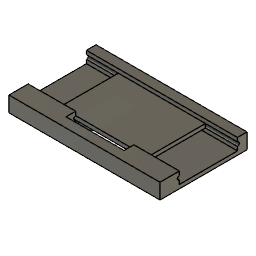
reaction wheel pendulum (Autodesk Fusion 360 archive; units mm, degrees)
design "computer stand"
Autodesk Fusion 360 part; units mm, degrees
(part 1 of 2)
sketch "スケッチ1" plane through (0, 0, 0) normal (0, 0, 1) x (1, 0, 0)
  line L0 (0, 0) -> (-50, 0)
  line L1 (-50, 0) -> (-50, -35)
  line L2 (-50, -35) -> (0, -35)
  line L3 (0, -35) -> (0, 0)
  line L4 (-65, 5) -> (15, 5)
  line L5 (15, 5) -> (15, -40)
  line L6 (15, -40) -> (-65, -40)
  line L7 (-65, -40) -> (-65, 5)
  constraint horizontal L0
  constraint vertical L1
  constraint horizontal L2
  constraint vertical L3
  constraint coincident L0.start L3.end
  constraint horizontal L4
  constraint vertical L5
  constraint horizontal L6
  constraint vertical L7
extrude "押し出し1" add sketch "スケッチ1" against normal blind 5 contours L0 L1 L2 L3 makes body 1
extrude "押し出し2" add sketch "スケッチ1" along normal blind 5 contours L0 L1 L2 L3 | L4 L5 L6 L7 bodies 1
sketch "スケッチ2" plane through (0, 0, 5) normal (0, 0, 1) x (-1, 0, 0)
  line L0 (65, 40) -> (-15, 40)
  line L1 (-15, 40) -> (-15, -5)
  line L2 (-15, -5) -> (65, -5)
  line L3 (65, -5) -> (65, 40)
  line L4 (-15, 0) -> (65, 0)
  line L5 (65, 0) -> (65, 30)
  line L6 (65, 30) -> (-15, 30)
  line L7 (-15, 30) -> (-15, 0)
  constraint horizontal L4
  constraint vertical L5
  constraint horizontal L6
  constraint vertical L7
  constraint coincident L3 L5.end
  constraint coincident L1 L4.start
extrude "押し出し3" cut sketch "スケッチ2" against normal blind 3 contours L1 L3 L4 L5 L6 L7 bodies 1
sketch "スケッチ3" plane through (0, 0, -5) normal (0, 0, -1) x (1, 0, 0)
  line L0 (0, 0) -> (0, 35)
  line L1 (0, 35) -> (-50, 35)
  line L2 (-50, 35) -> (-50, 0)
  line L3 (-50, 0) -> (0, 0)
  line L4 (-10, 0) -> (-40, 0)
  line L5 (-40, 0) -> (-40, 35)
  line L6 (-40, 35) -> (-10, 35)
  line L7 (-10, 35) -> (-10, 0)
  constraint horizontal L4
  constraint vertical L5
  constraint horizontal L6
  constraint vertical L7
  constraint coincident L1 L5.end
  constraint coincident L3 L4.start
extrude "押し出し4" cut sketch "スケッチ3" against normal blind 10 contours L1 L3 L4 L5 L6 L7 bodies 1
extrude "押し出し5" add 2 faces at (-38.3333, 3.3333, 5) (-56.6667, -35, 5) along direction (0, 0, 1) blind 3 on bodies 1 bodies 1
sketch "スケッチ4" plane through (-65, 0, 0) normal (-1, 0, 0) x (0, -1, 0)
  line L0 (0, 2) -> (0, 8)
  line L1 (0, 8) -> (-5, 8)
  line L2 (-5, 8) -> (-5, 0)
  line L3 (-5, 0) -> (40, 0)
  line L4 (40, 0) -> (40, 8)
  line L5 (40, 8) -> (30, 8)
  line L6 (30, 8) -> (30, 2)
  line L7 (30, 2) -> (0, 2)
  line L8 (0, 5) -> (30, 5)
  line L9 (0, 4) -> (30, 4)
  arc A0 (30, 4) -> (30, 6) centre (30, 5) ccw
  line L10 (30, 6) -> (0, 6)
  arc A1 (0, 6) -> (0, 4) centre (0, 5) ccw
  line L11 (0, 5) -> (30, 5) construction
  constraint midpoint L0 L8.start
  constraint midpoint L6 L8.end
  constraint tangent L9 A0
  constraint tangent A0 L10
  constraint parallel L9 L10
  constraint tangent L10 A1
  constraint tangent L9 A1
  constraint coincident L8.end A0.centre
  constraint perpendicular L6 L11
  constraint coincident L8.start A1.centre
extrude "押し出し6" cut sketch "スケッチ4" against normal blind 80 contours L0 A1 | L6 A0 bodies 1
sketch "スケッチ5" plane through (0, 0, -5) normal (0, 0, -1) x (1, 0, 0)
  line L0 (-40, 0) -> (-40, 35)
  line L1 (-40, 35) -> (-50, 35)
  line L2 (-50, 35) -> (-50, 0)
  line L3 (-50, 0) -> (-40, 0)
extrude "押し出し7" cut 1 faces at (-65, -36.9916, 4.2592) along direction (1, 0, 0) blind 1 on bodies 1 bodies 1
extrude "押し出し8" cut 1 faces at (-64, -36.9916, 4.2592) along direction (1, 0, 0) blind 1 on bodies 1 bodies 1
extrude "押し出し9" cut 1 faces at (15, -36.9916, 4.2592) along direction (-1, 0, 0) blind 1 on bodies 1 bodies 1
extrude "押し出し10" add 1 faces at (-63, -36.9916, 4.2592) along direction (-1, 0, 0) blind 0.5 on bodies 1 bodies 1
extrude "押し出し11" cut 1 faces at (14, -36.9916, 4.2592) along direction (-1, 0, 0) blind 0.5 on bodies 1 bodies 1
extrude "押し出し12" cut 1 faces at (0, -23.3333, -3.3333) along direction (-1, 0, 0) blind 0.25 on bodies 1 bodies 1
extrude "押し出し13" cut 1 faces at (-50, -11.6667, -3.3333) along direction (1, 0, 0) blind 0.25 on bodies 1 bodies 1
extrude "押し出し14" add 1 faces at (-63.5, -36.9916, 4.2592) along direction (-1, 0, 0) blind 1 on bodies 1 bodies 1
sketch "スケッチ6" plane through (-64.5, 0, 0) normal (-1, 0, 0) x (0, -1, 0)
  arc A0 (0, 6) -> (0, 4) centre (0, 5) ccw
  line L0 (0, 6) -> (0, 8)
  line L1 (0, 8) -> (-5, 8)
  line L2 (-5, 8) -> (-5, 0)
  line L3 (-5, 0) -> (40, 0)
  line L4 (40, 0) -> (40, 8)
  line L5 (40, 8) -> (30, 8)
  line L6 (30, 8) -> (30, 6)
  arc A1 (30, 4) -> (30, 6) centre (30, 5) ccw
  line L7 (30, 4) -> (30, 2)
  line L8 (30, 2) -> (0, 2)
  line L9 (0, 2) -> (0, 4)
  line L10 (0, 6) -> (30, 6)
  line L11 (30, 6) -> (30, 4)
  line L12 (30, 4) -> (0, 4)
  line L13 (0, 4) -> (0, 6)
  line L14 (0, 6) -> (30, 4) construction
  line L15 (30, 6) -> (0, 4) construction
  point P0 (15, 5)
  constraint horizontal L10
  constraint perpendicular L10 L11
  constraint parallel L10 L12
  constraint parallel L11 L13
  constraint coincident L14 P0
  constraint coincident L15 P0
  constraint coincident A0.start L0.start
  constraint coincident A1.start L7.start
extrude "押し出し15" add sketch "スケッチ6" against normal blind 78 separate body contours L10 L11 L12 L13 makes body 2
sketch "スケッチ7" plane through (0, 0, 6) normal (0, 0, 1) x (-1, 0, 0)
  line L0 (64.5, 0) -> (64.5, 30)
  line L1 (64.5, 30) -> (-13.5, 30)
  line L2 (-13.5, 30) -> (-13.5, 0)
  line L3 (-13.5, 0) -> (64.5, 0)
  line L4 (3, 30) -> (48, 30)
  line L5 (48, 30) -> (48, 0)
  line L6 (48, 0) -> (3, 0)
  line L7 (3, 0) -> (3, 30)
  line L8 (3, 30) -> (48, 0) construction
  line L9 (48, 30) -> (3, 0) construction
  point P0 (25.5, 15)
  dimension "d31" = 39
  dimension "d32" = 45
  constraint horizontal L4
  constraint perpendicular L4 L5
  constraint parallel L4 L6
  constraint parallel L5 L7
  constraint coincident L8 P0
  constraint coincident L9 P0
  constraint coincident L1 L4.start
  constraint coincident L3 L6.end
  measures "d31" distance of L2 P0
  measures "d32" distance of L4.start L4.end
extrude "押し出し16" cut sketch "スケッチ7" against normal blind 2 contours L0 L1 L3 L5 | L1 L2 L3 L7 bodies 2

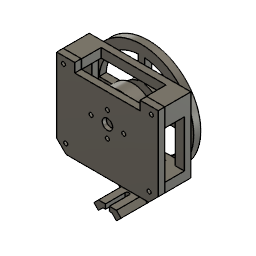
design "モータ取り付け台"
Autodesk Fusion 360 part; units mm, degrees
sketch "スケッチ1" plane through (0, 0, 0) normal (0, 0, 1) x (1, 0, 0)
  line L0 (-38.8909, 38.8909) -> (0, 0)
  line L1 (0, 0) -> (38.8909, 38.8909)
  line L2 (38.8909, 38.8909) -> (-38.8909, 38.8909) construction
  line L3 (0, 38.8909) -> (0, 0) construction
  line L4 (-24.5921, 31.6632) -> (-3.3789, 10.45)
  line L5 (-3.3789, 10.45) -> (3.3789, 10.45)
  line L6 (3.3789, 10.45) -> (24.5921, 31.6632)
  line L7 (24.5921, 31.6632) -> (24.5921, 38.8909)
  line L8 (-24.5921, 38.8909) -> (-24.5921, 31.6632)
  line L9 (-24.5921, 38.8909) -> (24.5921, 38.8909)
  line L10 (-38.8909, 38.8909) -> (-38.8909, 45.9909)
  line L11 (-31.8909, 45.9909) -> (31.8909, 45.9909)
  line L12 (38.8909, 45.9909) -> (38.8909, 38.8909)
  line L13 (31.8909, 45.9909) -> (-31.8909, 45.9909)
  line L14 (-38.8909, 45.9909) -> (-38.8909, 95.9909)
  line L15 (-38.8909, 95.9909) -> (38.8909, 95.9909)
  line L16 (38.8909, 95.9909) -> (38.8909, 45.9909)
  line L17 (38.8909, 45.9909) -> (-38.8909, 95.9909) construction
  line L18 (-38.8909, 45.9909) -> (38.8909, 95.9909) construction
  line L19 (-31.8909, 45.9909) -> (-31.8909, 81.9198)
  line L20 (-24.8198, 88.9909) -> (24.8198, 88.9909)
  line L21 (31.8909, 81.9198) -> (31.8909, 45.9909)
  line L22 (-24.8198, 88.9909) -> (-31.8909, 81.9198)
  line L23 (24.8198, 88.9909) -> (31.8909, 81.9198)
  point P0 (0, 70.9909)
  point P1 (0, 70.9909)
  dimension "d1" = 55
  dimension "d3" = 55
  dimension "d4" = 5
  dimension "d5" = 5
  dimension "d6" = 30
  dimension "d7" = 30
  dimension "d8" = 10.45
  dimension "d9" = 7.1
  dimension "d10" = 50
  dimension "d11" = 7
  dimension "d13" = 45
  dimension "d14" = 45
  dimension "d15" = 10
  dimension "d16" = 10
  dimension "d17" = 7
  dimension "d18" = 7
  dimension "d19" = 57.1
  dimension "d20" = 7.1
  constraint coincident L0.end L1.start
  constraint horizontal L2
  constraint midpoint L2 L3.start
  constraint perpendicular L3 L5
  constraint parallel L0 L4
  constraint parallel L1 L6
  constraint perpendicular L0 L1
  constraint vertical L8
  constraint vertical L7
  constraint coincident L2 L8.start
  constraint coincident L2 L7.end
  constraint coincident L0.start L2.end
  constraint horizontal L11
  constraint vertical L10
  constraint vertical L12
  constraint horizontal L13
  constraint perpendicular L13 L14
  constraint parallel L13 L15
  constraint parallel L14 L16
  constraint coincident L17 P1
  constraint coincident L18 P1
  constraint coincident L10.end L14.start
  constraint coincident P1 P0
  measures "d1" distance of L0.end L1.end
  measures "d3" distance of L0.start L0.end
  measures "d4" distance of L1 L6
  measures "d5" distance of L0 L4
  measures "d6" distance of L5.end L6.end
  measures "d7" distance of L4.start L4.end
  measures "d8" distance of L0.end L5
  measures "d9" distance of L9 L11
  measures "d10" distance of L12.start L15.end
  measures "d11" distance of L16 L21
  measures "d13" angle of L20 L22
  measures "d14" angle of L20 L23
  measures "d15" distance of L20.start L19.end
  measures "d16" distance of L20.end L21.start
  measures "d17" distance of L15 L20
  measures "d18" distance of L14 L19
  measures "d19" distance of L9 L15
  measures "d20" distance of L0.start L10.end
extrude "押し出し1" add sketch "スケッチ1" along normal mid plane 5 makes body 1
sketch "スケッチ2" plane through (0, 0, 2.5) normal (0, 0, 1) x (1, 0, 0)
  line L0 (-31.8909, 81.9198) -> (-24.8198, 88.9909)
  line L1 (-24.8198, 88.9909) -> (24.8198, 88.9909)
  line L2 (24.8198, 88.9909) -> (31.8909, 81.9198)
  line L3 (31.8909, 81.9198) -> (31.8909, 45.9909)
  line L4 (31.8909, 45.9909) -> (-31.8909, 45.9909)
  line L5 (-31.8909, 45.9909) -> (-31.8909, 81.9198)
  line L6 (-3.3789, 10.45) -> (-24.5921, 31.6632)
  line L7 (-24.5921, 31.6632) -> (-24.5921, 38.8909)
  line L8 (-24.5921, 38.8909) -> (24.5921, 38.8909)
  line L9 (24.5921, 38.8909) -> (24.5921, 31.6632)
  line L10 (24.5921, 31.6632) -> (3.3789, 10.45)
  line L11 (3.3789, 10.45) -> (-3.3789, 10.45)
  line L12 (-38.8909, 38.8909) -> (0, 0)
  line L13 (0, 0) -> (38.8909, 38.8909)
  line L14 (38.8909, 38.8909) -> (38.8909, 95.9909)
  line L15 (38.8909, 95.9909) -> (-38.8909, 95.9909)
  line L16 (-38.8909, 95.9909) -> (-38.8909, 38.8909)
  line L17 (-24.8198, 95.9909) -> (-24.8198, 88.9909)
  line L18 (-24.8198, 88.9909) -> (-31.8909, 81.9198)
  line L19 (-31.8909, 81.9198) -> (-38.8909, 81.9198)
  line L20 (-38.8909, 81.9198) -> (-38.8909, 95.9909)
  line L21 (-38.8909, 95.9909) -> (-24.8198, 95.9909)
  line L22 (24.8198, 95.9909) -> (24.8198, 88.9909)
  line L23 (24.8198, 88.9909) -> (31.8909, 81.9198)
  line L24 (31.8909, 81.9198) -> (38.8909, 81.9198)
  line L25 (38.8909, 81.9198) -> (38.8909, 95.9909)
  line L26 (38.8909, 95.9909) -> (24.8198, 95.9909)
  line L27 (-24.5921, 45.9909) -> (-24.5921, 31.6632)
  line L28 (-24.5921, 31.6632) -> (-31.6632, 31.6632)
  line L29 (-31.6632, 31.6632) -> (-38.8909, 38.8909)
  line L30 (-38.8909, 38.8909) -> (-38.8909, 45.9909)
  line L31 (-38.8909, 45.9909) -> (-24.5921, 45.9909)
  line L32 (24.5921, 45.9909) -> (24.5921, 31.6632)
  line L33 (24.5921, 31.6632) -> (31.6632, 31.6632)
  line L34 (31.6632, 31.6632) -> (38.8909, 38.8909)
  line L35 (38.8909, 38.8909) -> (38.8909, 45.9909)
  line L36 (38.8909, 45.9909) -> (24.5921, 45.9909)
  line L37 (-3.3789, 10.45) -> (-6.9145, 6.9145)
  line L38 (-6.9145, 6.9145) -> (0, 0)
  line L39 (0, 0) -> (6.9145, 6.9145)
  line L40 (6.9145, 6.9145) -> (3.3789, 10.45)
  line L41 (3.3789, 10.45) -> (-3.3789, 10.45)
  constraint coincident L15 L17.start
  constraint coincident L0.end L1.start
  constraint perpendicular L1 L17
  constraint coincident L0.start L5.end
  constraint coincident L16 L19.end
  constraint perpendicular L16 L19
  constraint coincident L15.end L16.start
  constraint coincident L15 L22.start
  constraint coincident L1.end L2.start
  constraint coincident L2.end L3.start
  constraint coincident L14 L24.end
  constraint perpendicular L14 L24
  constraint coincident L14.end L15.start
  constraint vertical L22
  constraint coincident L4 L27.start
  constraint coincident L6.end L7.start
  constraint coincident L12 L28.end
  constraint perpendicular L27 L28
  constraint vertical L27
  constraint coincident L16 L30.end
  constraint coincident L12.start L16.end
  constraint horizontal L31
  constraint vertical L32
  constraint perpendicular L32 L33
  constraint perpendicular L33 L35
  constraint coincident L4 L32.start
  constraint coincident L9.end L10.start
  constraint coincident L13 L33.end
  constraint coincident L14 L35.end
  constraint coincident L13.end L14.start
  constraint horizontal L36
  constraint coincident L6.start L11.end
  constraint coincident L12 L37.end
  constraint perpendicular L12 L37
  constraint perpendicular L12 L39
  constraint coincident L10.end L11.start
  constraint coincident L13 L39.end
  constraint coincident L12.end L13.start
  constraint perpendicular L13 L40
extrude "押し出し2" add sketch "スケッチ2" along normal blind 15 contours L0 L15 L16 L17 L18 L19 L20 L21 | L4 L7 L12 L16 L27 L28 L29 L30 L31 | L2 L14 L15 L22 L23 L24 L25 L26 | L4 L9 L13 L14 L32 L33 L34 L35 L36 bodies 1
extrude "押し出し3" add sketch "スケッチ2" along normal blind 60 contours L11 L12 L13 L37 L38 L39 L40 L41 bodies 1
sketch "スケッチ3" plane through (0, 0, -2.5) normal (0, 0, -1) x (-1, 0, 0)
  line L0 (24.8198, 88.9909) -> (31.8909, 81.9198)
  line L1 (31.8909, 81.9198) -> (31.8909, 45.9909)
  line L2 (31.8909, 45.9909) -> (-31.8909, 45.9909)
  line L3 (-31.8909, 45.9909) -> (-31.8909, 81.9198)
  line L4 (-31.8909, 81.9198) -> (-24.8198, 88.9909)
  line L5 (-24.8198, 88.9909) -> (24.8198, 88.9909)
  line L6 (24.5921, 31.6632) -> (3.3789, 10.45)
  line L7 (3.3789, 10.45) -> (-3.3789, 10.45)
  line L8 (-3.3789, 10.45) -> (-24.5921, 31.6632)
  line L9 (-24.5921, 31.6632) -> (-24.5921, 38.8909)
  line L10 (-24.5921, 38.8909) -> (24.5921, 38.8909)
  line L11 (24.5921, 38.8909) -> (24.5921, 31.6632)
  line L12 (0, 0) -> (38.8909, 38.8909)
  line L13 (38.8909, 38.8909) -> (38.8909, 95.9909)
  line L14 (38.8909, 95.9909) -> (-38.8909, 95.9909)
  line L15 (-38.8909, 95.9909) -> (-38.8909, 38.8909)
  line L16 (-38.8909, 38.8909) -> (0, 0)
  line L17 (-38.8909, 95.9909) -> (-28.3553, 85.4553) construction
  line L18 (38.8909, 95.9909) -> (28.3553, 85.4553) construction
  circle A0 centre (-33.6231, 90.7231) radius 3.5
  circle A1 centre (33.6231, 90.7231) radius 3.5
  circle A2 centre (-31.8909, 38.8909) radius 3.5
  circle A3 centre (31.8909, 38.8909) radius 3.5
  line L19 (-24.5921, 38.8909) -> (-38.8909, 38.8909) construction
  line L20 (-31.8909, 45.9909) -> (-31.8909, 31.8909) construction
  line L21 (24.5921, 38.8909) -> (38.8909, 38.8909) construction
  line L22 (31.8909, 45.9909) -> (31.8909, 31.8909) construction
  circle A4 centre (-31.8909, 38.8909) radius 1.5
  circle A5 centre (31.8909, 38.8909) radius 1.5
  circle A6 centre (33.6231, 90.7231) radius 1.5
  circle A7 centre (-33.6231, 90.7231) radius 1.5
  dimension "d27" = 7
  dimension "d28" = 7
  dimension "d29" = 7
  dimension "d30" = 7
  dimension "d31" = 3
  dimension "d32" = 3
  dimension "d33" = 3
  dimension "d34" = 3
  constraint coincident L14.end L15.start
  constraint midpoint L4 L17.end
  constraint coincident L13.end L14.start
  constraint midpoint L0 L18.end
  constraint midpoint L17 A0.centre
  constraint midpoint L18 A1.centre
  constraint coincident L9.end L10.start
  constraint coincident L15.end L16.start
  constraint coincident L2.end L3.start
  constraint coincident L16 L20.end
  constraint perpendicular L19 L20
  constraint coincident A2.centre L19
  constraint coincident A2.centre L20
  constraint coincident L10.end L11.start
  constraint coincident L12.end L13.start
  constraint coincident L1.end L2.start
  constraint coincident L12 L22.end
  constraint perpendicular L21 L22
  constraint coincident A3.centre L22
  constraint coincident A3.centre L21
  constraint concentric A2 A4
  constraint concentric A3 A5
  constraint concentric A1 A6
  constraint concentric A0 A7
  measures "d27" diameter of A0
  measures "d28" diameter of A1
  measures "d29" diameter of A2
  measures "d30" diameter of A3
  measures "d31" diameter of A4
  measures "d32" diameter of A5
  measures "d33" diameter of A6
  measures "d34" diameter of A7
extrude "押し出し4" cut sketch "スケッチ3" against normal blind 25 contours A4 | A5 | A6 | A7 bodies 1
extrude "押し出し7" cut 1 faces at (0, 6.9667, 62.5) along direction (0, 0, -1) blind 65 on bodies 1 bodies 1
sketch "スケッチ8" plane through (0, 0, 2.5) normal (0, 0, 1) x (1, 0, 0)
  line L0 (-6.9145, 6.9145) -> (-3.3789, 10.45)
  line L1 (-3.3789, 10.45) -> (-24.5921, 31.6632)
  line L2 (-24.5921, 31.6632) -> (-31.6632, 31.6632)
  line L3 (-31.6632, 31.6632) -> (-6.9145, 6.9145)
  line L4 (3.3789, 10.45) -> (6.9145, 6.9145)
  line L5 (24.5921, 31.6632) -> (3.3789, 10.45)
  line L6 (6.9145, 6.9145) -> (31.6632, 31.6632)
  line L7 (-3.3789, 10.45) -> (3.3789, 10.45)
  line L8 (-6.9145, 13.9855) -> (6.9145, 13.9855)
  line L9 (6.9145, 13.9855) -> (10.45, 10.45)
  line L10 (-6.9145, 13.9855) -> (-10.45, 10.45)
  dimension "d52" = 5
  dimension "d53" = 5
  constraint coincident L0.end L1.start
  constraint coincident L4.start L5.end
  constraint coincident L1 L8.start
  constraint coincident L5 L8.end
  constraint coincident L6 L9.end
  constraint coincident L3 L10.end
  constraint perpendicular L1 L10
  constraint perpendicular L6 L9
  measures "d52" distance of L0 L10
  measures "d53" distance of L4 L9
extrude "押し出し9" add sketch "スケッチ8" against normal blind 5 contours L1 L5 L7 L8 bodies 1
extrude "押し出し10" add sketch "スケッチ8" along normal blind 20 contours L0 L1 L3 L10 | L1 L5 L7 L8 | L4 L5 L6 L9 bodies 1
sketch "スケッチ9" plane through (0, 10.45, 0) normal (0, -1, 0) x (1, 0, 0)
  line L0 (-3.3789, 22.5) -> (-3.3789, -2.5)
  line L1 (-3.3789, -2.5) -> (3.3789, -2.5)
  line L2 (3.3789, -2.5) -> (3.3789, 22.5)
  line L3 (3.3789, 22.5) -> (-3.3789, 22.5)
  arc A0 (-1.5, 7.5) -> (1.5, 7.5) centre (0, 7.5) ccw
  line L4 (0, 7.5) -> (0, -2.5) construction
  line L5 (-1.5, 7.5) -> (-1.5, 22.5)
  line L6 (1.5, 22.5) -> (1.5, 7.5)
  dimension "d58" = 10
  dimension "d59" = 1.5
  constraint coincident A0.centre L4.start
  constraint midpoint L1 L4.end
  constraint vertical L4
  constraint coincident L3 L5.end
  constraint tangent A0 L5
  constraint coincident L3 L6.start
  constraint tangent A0 L6
  constraint vertical L6
  constraint vertical L5
  measures "d58" distance of A0.centre L4.end
  measures "d59" radius of A0
extrude "押し出し11" cut sketch "スケッチ9" against normal blind 4 contours L3 A0 L5 L6 bodies 1
extrude "押し出し12" add sketch "スケッチ3" against normal blind 4 contours A4 | A5 | A6 | A7 bodies 1
sketch "スケッチ10" plane through (0, 0, 17.5) normal (0, 0, 1) x (1, 0, 0)
  circle A0 centre (-31.8909, 38.8909) radius 1.5
  line L0 (-38.8909, 45.9909) -> (-38.8909, 38.8909)
  line L1 (-38.8909, 38.8909) -> (-31.6632, 31.6632)
  line L2 (-31.6632, 31.6632) -> (-24.5921, 31.6632)
  line L3 (-24.5921, 31.6632) -> (-24.5921, 45.9909)
  line L4 (-24.5921, 45.9909) -> (-38.8909, 45.9909)
  line L5 (-38.8909, 95.9909) -> (-38.8909, 81.9198)
  line L6 (31.6632, 31.6632) -> (38.8909, 38.8909)
  line L7 (38.8909, 81.9198) -> (38.8909, 95.9909)
  line L8 (-38.8909, 95.9909) -> (-38.8909, 38.8909)
  line L9 (-38.8909, 38.8909) -> (-31.6632, 31.6632)
  line L10 (-31.6632, 31.6632) -> (31.6632, 31.6632)
  line L11 (31.6632, 31.6632) -> (38.8909, 38.8909)
  line L12 (38.8909, 38.8909) -> (38.8909, 95.9909)
  line L13 (38.8909, 95.9909) -> (-38.8909, 95.9909)
  line L14 (31.8909, 45.9909) -> (31.8909, 81.9198)
  line L15 (31.8909, 81.9198) -> (24.8198, 88.9909)
  line L16 (6.9145, 13.9855) -> (24.5921, 31.6632)
  line L17 (24.5921, 31.6632) -> (24.5921, 38.8909)
  line L18 (24.5921, 38.8909) -> (-24.5921, 38.8909)
  line L19 (-24.5921, 38.8909) -> (-24.5921, 31.6632)
  line L20 (-24.5921, 31.6632) -> (-6.9145, 13.9855)
  line L21 (-6.9145, 13.9855) -> (6.9145, 13.9855)
  line L22 (3.3789, 10.45) -> (-3.3789, 10.45)
  line L23 (-3.3789, 10.45) -> (-6.9145, 6.9145)
  line L24 (-6.9145, 6.9145) -> (-38.8909, 38.8909)
  line L25 (-38.8909, 38.8909) -> (-38.8909, 95.9909)
  line L26 (-38.8909, 95.9909) -> (38.8909, 95.9909)
  line L27 (38.8909, 95.9909) -> (38.8909, 38.8909)
  line L28 (38.8909, 38.8909) -> (6.9145, 6.9145)
  line L29 (6.9145, 6.9145) -> (3.3789, 10.45)
  line L30 (-24.8198, 88.9909) -> (-31.8909, 81.9198)
  line L31 (-31.8909, 81.9198) -> (-31.8909, 45.9909)
  line L32 (-31.8909, 45.9909) -> (31.8909, 45.9909)
  line L33 (31.8909, 45.9909) -> (31.8909, 81.9198)
  line L34 (31.8909, 81.9198) -> (24.8198, 88.9909)
  line L35 (24.8198, 88.9909) -> (-24.8198, 88.9909)
  line L36 (0, 88.9909) -> (0, 45.9909) construction
  circle A1 centre (0, 76.9909) radius 1.5
  circle A2 centre (12.5, 67.4909) radius 1.5
  circle A3 centre (0, 57.9909) radius 1.5
  circle A4 centre (-12.5, 67.4909) radius 1.5
  line L37 (-12.5, 67.4909) -> (12.5, 67.4909) construction
  line L38 (0, 76.9909) -> (0, 57.9909) construction
  circle A5 centre (31.8909, 38.8909) radius 1.5
  circle A6 centre (33.6231, 90.7231) radius 1.5
  circle A7 centre (-33.6231, 90.7231) radius 1.5
  circle A8 centre (-33.6231, 90.7231) radius 1.5
  circle A9 centre (33.6231, 90.7231) radius 1.5
  circle A10 centre (31.8909, 38.8909) radius 1.5
  circle A11 centre (0, 67.4909) radius 4
  point P0 (0, 67.4909)
  dimension "d64" = 3
  dimension "d65" = 3
  dimension "d66" = 3
  dimension "d67" = 3
  dimension "d68" = 19
  dimension "d69" = 25
  dimension "d70" = 12.5
  dimension "d71" = 9.5
  dimension "d78" = 3
  dimension "d79" = 3
  dimension "d80" = 3
  dimension "d81" = 8
  constraint coincident L5.start L8.start
  constraint coincident L0.end L1.start
  constraint coincident L1.end L2.start
  constraint coincident L6.start L10.end
  constraint coincident L6.end L11.end
  constraint coincident L7.end L12.end
  constraint midpoint L35 L36.start
  constraint midpoint L32 L36.end
  constraint midpoint L36 P0
  constraint coincident A4.centre L37.start
  constraint coincident A2.centre L37.end
  constraint coincident A1.centre L38.start
  constraint coincident A3.centre L38.end
  constraint coincident P0 L37
  constraint coincident P0 L38
  constraint vertical L38
  constraint horizontal L37
  constraint concentric A7 A8
  constraint concentric A6 A9
  constraint concentric A5 A10
  constraint coincident P0 A11.centre
  measures "d64" diameter of A1
  measures "d65" diameter of A3
  measures "d66" diameter of A4
  measures "d67" diameter of A2
  measures "d68" distance of A1.centre A3.centre
  measures "d69" distance of A2.centre A4.centre
  measures "d70" distance of P0 A2.centre
  measures "d71" distance of P0 A1.centre
  measures "d78" diameter of A10
  measures "d79" diameter of A9
  measures "d80" diameter of A8
  measures "d81" diameter of A11
extrude "押し出し13" add sketch "スケッチ10" along normal blind 5 separate body contours L0 L1 L2 L3 L4 L8 L9 L10 L19 L24 L25 L32 | L3 L4 L5 L6 L7 L8 L10 L11 L12 L13 L14 L15 L17 L18 L25 L26 L27 L28 L30 L31 L32 L33 L34 L35 | L4 L14 L15 L30 L31 L32 L33 L34 L35 | L3 L10 L17 L18 L19 makes body 2
sketch "スケッチ11" plane through (0, 0, 22.5) normal (0, 0, 1) x (1, 0, 0)
  circle A0 centre (-12.5, 67.4909) radius 1.5
  circle A1 centre (0, 76.9909) radius 1.5
  circle A2 centre (0, 57.9909) radius 1.5
  circle A3 centre (12.5, 67.4909) radius 1.5
  line L0 (-31.6632, 31.6632) -> (31.6632, 31.6632)
  line L1 (31.6632, 31.6632) -> (38.8909, 38.8909)
  line L2 (38.8909, 38.8909) -> (38.8909, 95.9909)
  line L3 (38.8909, 95.9909) -> (-38.8909, 95.9909)
  line L4 (-38.8909, 95.9909) -> (-38.8909, 38.8909)
  line L5 (-38.8909, 38.8909) -> (-31.6632, 31.6632)
  line L6 (25, 95.9909) -> (-25, 95.9909)
  line L7 (-25, 95.9909) -> (-25, 88.9909)
  line L8 (-25, 88.9909) -> (25, 88.9909)
  line L9 (25, 88.9909) -> (25, 95.9909)
  line L10 (25, 95.9909) -> (-25, 88.9909) construction
  line L11 (-25, 95.9909) -> (25, 88.9909) construction
  line L12 (0, 76.9909) -> (0, 92.4909) construction
  circle A4 centre (-31.8909, 38.8909) radius 1.5
  circle A5 centre (31.8909, 38.8909) radius 1.5
  circle A6 centre (33.6231, 90.7231) radius 1.5
  circle A7 centre (-33.6231, 90.7231) radius 1.5
  circle A8 centre (0, 67.4909) radius 4
  point P0 (0, 92.4909)
  dimension "d74" = 50
  dimension "d75" = 7
  constraint horizontal L6
  constraint perpendicular L6 L7
  constraint parallel L6 L8
  constraint parallel L7 L9
  constraint coincident L10 P0
  constraint coincident L11 P0
  constraint coincident L3 L6.start
  constraint coincident A1.centre L12.start
  constraint coincident P0 L12.end
  constraint vertical L12
  measures "d74" distance of L7.end L8.end
  measures "d75" distance of L6.start L8.end
extrude "押し出し14" cut sketch "スケッチ11" against normal blind 5 contours L3 L6 L7 L8 L9 bodies 2
sketch "スケッチ12" plane through (0, 0, 17.5) normal (0, 0, -1) x (-1, 0, 0)
  line L0 (25, 95.9909) -> (25, 88.9909)
  line L1 (25, 88.9909) -> (-25, 88.9909)
  line L2 (-25, 88.9909) -> (-25, 95.9909)
  line L3 (-25, 95.9909) -> (-38.8909, 95.9909)
  line L4 (-38.8909, 95.9909) -> (-38.8909, 38.8909)
  line L5 (-38.8909, 38.8909) -> (-31.6632, 31.6632)
  line L6 (-31.6632, 31.6632) -> (31.6632, 31.6632)
  line L7 (31.6632, 31.6632) -> (38.8909, 38.8909)
  line L8 (38.8909, 38.8909) -> (38.8909, 95.9909)
  line L9 (38.8909, 95.9909) -> (25, 95.9909)
  circle A0 centre (-12.5, 67.4909) radius 1.5
  circle A1 centre (0, 57.9909) radius 1.5
  circle A2 centre (33.6231, 90.7231) radius 1.5
  circle A3 centre (0, 67.4909) radius 4
  circle A4 centre (-31.8909, 38.8909) radius 1.5
  circle A5 centre (31.8909, 38.8909) radius 1.5
  circle A6 centre (12.5, 67.4909) radius 1.5
  circle A7 centre (-33.6231, 90.7231) radius 1.5
  circle A8 centre (0, 76.9909) radius 1.5
  circle A9 centre (0, 67.4909) radius 16.25
  dimension "d82" = 32.5
  constraint concentric A3 A9
  measures "d82" diameter of A9
extrude "押し出し15" add sketch "スケッチ12" along normal blind 1.5 separate body contours A9 makes body 3
sketch "スケッチ13" plane through (0, 0, 16) normal (0, 0, -1) x (-1, 0, 0)
  circle A0 centre (0, 76.9909) radius 1.5
  circle A1 centre (0, 67.4909) radius 4
  circle A2 centre (0, 57.9909) radius 1.5
  circle A3 centre (12.5, 67.4909) radius 1.5
  circle A4 centre (-12.5, 67.4909) radius 1.5
  circle A5 centre (0, 67.4909) radius 16.25
  circle A6 centre (0, 67.4909) radius 7.5
  dimension "d85" = 15
  constraint concentric A1 A6
  measures "d85" diameter of A6
extrude "押し出し16" add sketch "スケッチ13" along normal blind 3 contours A6 bodies 3
sketch "スケッチ15" plane through (0, 0, 13) normal (0, 0, -1) x (-1, 0, 0)
  circle A0 centre (0, 67.4909) radius 4
  circle A1 centre (0, 67.4909) radius 7.5
  circle A2 centre (0, 67.4909) radius 17.5
  dimension "d88" = 35
  constraint concentric A0 A2
  measures "d88" diameter of A2
extrude "押し出し17" add sketch "スケッチ15" along normal blind 9 contours A0 | A1 | A2 bodies 3
sketch "スケッチ16" plane through (0, 0, 13) normal (0, 0, 1) x (1, 0, 0)
  circle A0 centre (0, 67.4909) radius 4
  circle A1 centre (0, 67.4909) radius 3.25
  dimension "d91" = 6.5
  constraint concentric A0 A1
  measures "d91" diameter of A1
extrude "押し出し18" add sketch "スケッチ16" along normal blind 7 contours A1 bodies 3
sketch "スケッチ17" plane through (0, 0, 0) normal (1, 0, 0) x (0, 0, -1)
  line L0 (-4, 49.9909) -> (-4, 84.9909)
  line L1 (-4, 84.9909) -> (-3, 84.9909)
  line L2 (-18, 67.4909) -> (2, 67.4909)
  line L3 (-1, 67.4909) -> (-4, 67.4909)
  line L4 (-4, 84.9909) -> (-4, 67.4909)
  line L5 (-20, 70.7409) -> (-20, 64.2409)
  line L6 (-3, 84.9909) -> (-1, 74.4909)
  line L7 (-1, 74.4909) -> (-1, 67.4909)
  dimension "d94" = 19
  dimension "d95" = 1
  dimension "d96" = 7
  constraint coincident L0.end L1.start
  constraint perpendicular L0 L1
  constraint coincident L3.start L2
  constraint midpoint L0 L3.end
  constraint vertical L7
  measures "d94" distance of L3.start L5
  measures "d95" distance of L0.end L1.end
  measures "d96" distance of L3.start L6.end
revolve "回転1" add sketch "スケッチ17" angle 360 about axis through (0, 67.4909, 18) along (0, 0, -1) bodies 3
sketch "スケッチ18" plane through (0, 0, 1) normal (0, 0, -1) x (-1, 0, 0)
  circle A0 centre (0, 67.4909) radius 7
  circle A1 centre (0, 67.4909) radius 2
  dimension "d98" = 4
  constraint concentric A0 A1
  measures "d98" diameter of A1
extrude "押し出し19" add sketch "スケッチ18" along normal blind 9.1 contours A1 bodies 3
sketch "スケッチ19" plane through (0, 0, -2.5) normal (0, 0, -1) x (-1, 0, 0)
  line L0 (-6.9145, 13.9855) -> (-24.5921, 31.6632)
  line L1 (-24.5921, 31.6632) -> (-24.5921, 38.8909)
  line L2 (-24.5921, 38.8909) -> (24.5921, 38.8909)
  line L3 (24.5921, 38.8909) -> (24.5921, 31.6632)
  line L4 (24.5921, 31.6632) -> (6.9145, 13.9855)
  line L5 (6.9145, 13.9855) -> (-6.9145, 13.9855)
  line L6 (-3.3789, 10.45) -> (3.3789, 10.45)
  line L7 (3.3789, 10.45) -> (6.9145, 6.9145)
  line L8 (6.9145, 6.9145) -> (38.8909, 38.8909)
  line L9 (38.8909, 38.8909) -> (38.8909, 95.9909)
  line L10 (38.8909, 95.9909) -> (-38.8909, 95.9909)
  line L11 (-38.8909, 95.9909) -> (-38.8909, 38.8909)
  line L12 (-38.8909, 38.8909) -> (-6.9145, 6.9145)
  line L13 (-6.9145, 6.9145) -> (-3.3789, 10.45)
  line L14 (24.8198, 88.9909) -> (31.8909, 81.9198)
  line L15 (31.8909, 81.9198) -> (31.8909, 45.9909)
  line L16 (31.8909, 45.9909) -> (-31.8909, 45.9909)
  line L17 (-31.8909, 45.9909) -> (-31.8909, 81.9198)
  line L18 (-31.8909, 81.9198) -> (-24.8198, 88.9909)
  line L19 (-24.8198, 88.9909) -> (24.8198, 88.9909)
  circle A0 centre (0, 67.4909) radius 2
  circle A1 centre (0, 67.4909) radius 2
  circle A2 centre (0, 67.4909) radius 40
  circle A3 centre (0, 67.4909) radius 15
  circle A4 centre (0, 67.4909) radius 3.75
  circle A5 centre (0, 67.4909) radius 32.5
  line L20 (-2.5, 99.8946) -> (-2.5, 82.2811)
  line L21 (2.5, 99.8946) -> (2.5, 82.2811)
  line L22 (14.7902, 69.9909) -> (32.4037, 69.9909)
  line L23 (14.7902, 64.9909) -> (32.4037, 64.9909)
  line L24 (2.5, 52.7007) -> (2.5, 35.0872)
  line L25 (-2.5, 52.7007) -> (-2.5, 35.0872)
  line L26 (-14.7902, 64.9909) -> (-32.4037, 64.9909)
  line L27 (-14.7902, 69.9909) -> (-32.4037, 69.9909)
  dimension "d101" = 4
  dimension "d102" = 80
  dimension "d103" = 30
  dimension "d104" = 7.5
  dimension "d107" = 65
  dimension "d108" = 5
  dimension "d109" = 5
  dimension "d110" = 5
  dimension "d111" = 5
  dimension "d112" = 2.5
  dimension "d113" = 2.5
  dimension "d114" = 2.5
  dimension "d115" = 2.5
  constraint concentric A0 A1
  constraint concentric A0 A2
  constraint concentric A1 A3
  constraint concentric A3 A4
  constraint concentric A1 A5
  constraint coincident A5 L20.start
  constraint coincident A3 L20.end
  constraint perpendicular L19 L20
  constraint coincident A5 L21.start
  constraint coincident A3 L21.end
  constraint perpendicular L19 L21
  constraint coincident A3 L22.start
  constraint coincident A5 L22.end
  constraint perpendicular L15 L22
  constraint coincident A3 L23.start
  constraint coincident A3 L24.start
  constraint coincident A5 L24.end
  constraint perpendicular L2 L24
  constraint coincident A3 L25.start
  constraint coincident A5 L25.end
  constraint coincident A3 L26.start
  constraint coincident A5 L26.end
  constraint coincident A3 L27.start
  constraint coincident A5 L27.end
  constraint coincident A5 L23.end
  constraint horizontal L27
  constraint horizontal L26
  constraint horizontal L23
  constraint vertical L25
  measures "d101" diameter of A1
  measures "d102" diameter of A2
  measures "d103" diameter of A3
  measures "d104" diameter of A4
  measures "d107" diameter of A5
  measures "d108" distance of L22 L23
  measures "d109" distance of L20 L21
  measures "d110" distance of L26 L27
  measures "d111" distance of L24 L25
  measures "d112" distance of A0.centre L27
  measures "d113" distance of A0.centre L21
  measures "d114" distance of A0.centre L22
  measures "d115" distance of A0.centre L24
extrude "押し出し20" add sketch "スケッチ19" against normal blind 3.5 separate body contours A4 makes body 4
extrude "押し出し21" add sketch "スケッチ19" along normal blind 6.5 contours L1 L2 L10 L11 L16 L17 L18 L19 A2 A5 | L1 L2 L3 A2 A5 | L11 A2 | L2 L3 L9 L10 L14 L15 L16 L19 A2 A5 | L9 A2 | L2 L16 L24 L25 | L2 A5 L24 L25 | L16 L17 A5 | L10 A2 A5 | L16 A3 L24 L25 | L15 L16 A5 | A3 | L17 A5 L26 L27 | L17 A3 L26 L27 | L10 A5 L20 L21 | L10 L19 L20 L21 | L17 L18 L19 A5 | L19 A3 L20 L21 | L14 L15 L19 A5 | L15 A3 L22 L23 | L15 A5 L22 L23 | A4 bodies 4
extrude "押し出し22" cut 1 faces at (26.5325, 68.3242, -2.5) along direction (0, 0, -1) blind 1 on bodies 4 bodies 4
sketch "スケッチ20" plane through (0, 0, -9) normal (0, 0, -1) x (-1, 0, 0)
  circle A0 centre (0, 67.4909) radius 2
  line L0 (32.4037, 69.9909) -> (14.7902, 69.9909)
  arc A1 (14.7902, 69.9909) -> (2.5, 82.2811) centre (0, 67.4909) ccw
  line L1 (2.5, 82.2811) -> (2.5, 99.8946)
  arc A2 (32.4037, 69.9909) -> (2.5, 99.8946) centre (0, 67.4909) ccw
  arc A3 (-2.5, 99.8946) -> (-32.4037, 69.9909) centre (0, 67.4909) ccw
  line L2 (-2.5, 99.8946) -> (-2.5, 82.2811)
  arc A4 (-2.5, 82.2811) -> (-14.7902, 69.9909) centre (0, 67.4909) ccw
  line L3 (-14.7902, 69.9909) -> (-32.4037, 69.9909)
  arc A5 (2.5, 52.7007) -> (14.7902, 64.9909) centre (0, 67.4909) ccw
  line L4 (14.7902, 64.9909) -> (32.4037, 64.9909)
  arc A6 (2.5, 35.0872) -> (32.4037, 64.9909) centre (0, 67.4909) ccw
  line L5 (2.5, 35.0872) -> (2.5, 52.7007)
  arc A7 (-14.7902, 64.9909) -> (-2.5, 52.7007) centre (0, 67.4909) ccw
  line L6 (-2.5, 52.7007) -> (-2.5, 35.0872)
  arc A8 (-32.4037, 64.9909) -> (-2.5, 35.0872) centre (0, 67.4909) ccw
  line L7 (-32.4037, 64.9909) -> (-14.7902, 64.9909)
  circle A9 centre (0, 67.4909) radius 40
  circle A10 centre (0, 67.4909) radius 2
  dimension "d120" = 4
  constraint concentric A0 A10
  measures "d120" diameter of A10
extrude "押し出し23" add sketch "スケッチ20" against normal blind 0.9 contours A0 A10 bodies 4
named bodies: "モータ取り付け台", "BLDC", "リアクションホイール"

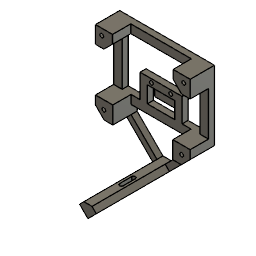
design "土台1(new)"
Autodesk Fusion 360 part; units mm, degrees
sketch "スケッチ1" plane through (0, 0, 0) normal (0, 0, 1) x (1, 0, 0)
  line L0 (-38.8909, 38.8909) -> (0, 0)
  line L1 (0, 0) -> (38.8909, 38.8909)
  line L2 (38.8909, 38.8909) -> (-38.8909, 38.8909) construction
  line L3 (0, 38.8909) -> (0, 0) construction
  line L4 (-24.5921, 31.6632) -> (-3.3789, 10.45)
  line L5 (-3.3789, 10.45) -> (3.3789, 10.45)
  line L6 (3.3789, 10.45) -> (24.5921, 31.6632)
  line L7 (24.5921, 31.6632) -> (24.5921, 38.8909)
  line L8 (-24.5921, 38.8909) -> (-24.5921, 31.6632)
  line L9 (-24.5921, 38.8909) -> (24.5921, 38.8909)
  line L10 (-38.8909, 38.8909) -> (-38.8909, 45.9909)
  line L11 (-31.8909, 45.9909) -> (31.8909, 45.9909)
  line L12 (38.8909, 45.9909) -> (38.8909, 38.8909)
  line L13 (31.8909, 45.9909) -> (-31.8909, 45.9909)
  line L14 (-38.8909, 45.9909) -> (-38.8909, 95.9909)
  line L15 (-38.8909, 95.9909) -> (38.8909, 95.9909)
  line L16 (38.8909, 95.9909) -> (38.8909, 45.9909)
  line L17 (38.8909, 45.9909) -> (-38.8909, 95.9909) construction
  line L18 (-38.8909, 45.9909) -> (38.8909, 95.9909) construction
  line L19 (-31.8909, 45.9909) -> (-31.8909, 81.9198)
  line L20 (-24.8198, 88.9909) -> (24.8198, 88.9909)
  line L21 (31.8909, 81.9198) -> (31.8909, 45.9909)
  line L22 (-24.8198, 88.9909) -> (-31.8909, 81.9198)
  line L23 (24.8198, 88.9909) -> (31.8909, 81.9198)
  point P0 (0, 70.9909)
  point P1 (0, 70.9909)
  dimension "d1" = 55
  dimension "d3" = 55
  dimension "d4" = 5
  dimension "d5" = 5
  dimension "d6" = 30
  dimension "d7" = 30
  dimension "d8" = 10.45
  dimension "d9" = 7.1
  dimension "d10" = 50
  dimension "d11" = 7
  dimension "d13" = 45
  dimension "d14" = 45
  dimension "d15" = 10
  dimension "d16" = 10
  dimension "d17" = 7
  dimension "d18" = 7
  dimension "d19" = 57.1
  dimension "d20" = 7.1
  constraint coincident L0.end L1.start
  constraint horizontal L2
  constraint midpoint L2 L3.start
  constraint perpendicular L3 L5
  constraint parallel L0 L4
  constraint parallel L1 L6
  constraint perpendicular L0 L1
  constraint vertical L8
  constraint vertical L7
  constraint coincident L2 L8.start
  constraint coincident L2 L7.end
  constraint coincident L0.start L2.end
  constraint horizontal L11
  constraint vertical L10
  constraint vertical L12
  constraint horizontal L13
  constraint perpendicular L13 L14
  constraint parallel L13 L15
  constraint parallel L14 L16
  constraint coincident L17 P1
  constraint coincident L18 P1
  constraint coincident L10.end L14.start
  constraint coincident P1 P0
  measures "d1" distance of L0.end L1.end
  measures "d3" distance of L0.start L0.end
  measures "d4" distance of L1 L6
  measures "d5" distance of L0 L4
  measures "d6" distance of L5.end L6.end
  measures "d7" distance of L4.start L4.end
  measures "d8" distance of L0.end L5
  measures "d9" distance of L9 L11
  measures "d10" distance of L12.start L15.end
  measures "d11" distance of L16 L21
  measures "d13" angle of L20 L22
  measures "d14" angle of L20 L23
  measures "d15" distance of L20.start L19.end
  measures "d16" distance of L20.end L21.start
  measures "d17" distance of L15 L20
  measures "d18" distance of L14 L19
  measures "d19" distance of L9 L15
  measures "d20" distance of L0.start L10.end
extrude "押し出し1" add sketch "スケッチ1" along normal mid plane 5 makes body 1
sketch "スケッチ2" plane through (0, 0, 2.5) normal (0, 0, 1) x (1, 0, 0)
  line L0 (-31.8909, 81.9198) -> (-24.8198, 88.9909)
  line L1 (-24.8198, 88.9909) -> (24.8198, 88.9909)
  line L2 (24.8198, 88.9909) -> (31.8909, 81.9198)
  line L3 (31.8909, 81.9198) -> (31.8909, 45.9909)
  line L4 (31.8909, 45.9909) -> (-31.8909, 45.9909)
  line L5 (-31.8909, 45.9909) -> (-31.8909, 81.9198)
  line L6 (-3.3789, 10.45) -> (-24.5921, 31.6632)
  line L7 (-24.5921, 31.6632) -> (-24.5921, 38.8909)
  line L8 (-24.5921, 38.8909) -> (24.5921, 38.8909)
  line L9 (24.5921, 38.8909) -> (24.5921, 31.6632)
  line L10 (24.5921, 31.6632) -> (3.3789, 10.45)
  line L11 (3.3789, 10.45) -> (-3.3789, 10.45)
  line L12 (-38.8909, 38.8909) -> (0, 0)
  line L13 (0, 0) -> (38.8909, 38.8909)
  line L14 (38.8909, 38.8909) -> (38.8909, 95.9909)
  line L15 (38.8909, 95.9909) -> (-38.8909, 95.9909)
  line L16 (-38.8909, 95.9909) -> (-38.8909, 38.8909)
  line L17 (-24.8198, 95.9909) -> (-24.8198, 88.9909)
  line L18 (-24.8198, 88.9909) -> (-31.8909, 81.9198)
  line L19 (-31.8909, 81.9198) -> (-38.8909, 81.9198)
  line L20 (-38.8909, 81.9198) -> (-38.8909, 95.9909)
  line L21 (-38.8909, 95.9909) -> (-24.8198, 95.9909)
  line L22 (24.8198, 95.9909) -> (24.8198, 88.9909)
  line L23 (24.8198, 88.9909) -> (31.8909, 81.9198)
  line L24 (31.8909, 81.9198) -> (38.8909, 81.9198)
  line L25 (38.8909, 81.9198) -> (38.8909, 95.9909)
  line L26 (38.8909, 95.9909) -> (24.8198, 95.9909)
  line L27 (-24.5921, 45.9909) -> (-24.5921, 31.6632)
  line L28 (-24.5921, 31.6632) -> (-31.6632, 31.6632)
  line L29 (-31.6632, 31.6632) -> (-38.8909, 38.8909)
  line L30 (-38.8909, 38.8909) -> (-38.8909, 45.9909)
  line L31 (-38.8909, 45.9909) -> (-24.5921, 45.9909)
  line L32 (24.5921, 45.9909) -> (24.5921, 31.6632)
  line L33 (24.5921, 31.6632) -> (31.6632, 31.6632)
  line L34 (31.6632, 31.6632) -> (38.8909, 38.8909)
  line L35 (38.8909, 38.8909) -> (38.8909, 45.9909)
  line L36 (38.8909, 45.9909) -> (24.5921, 45.9909)
  line L37 (-3.3789, 10.45) -> (-6.9145, 6.9145)
  line L38 (-6.9145, 6.9145) -> (0, 0)
  line L39 (0, 0) -> (6.9145, 6.9145)
  line L40 (6.9145, 6.9145) -> (3.3789, 10.45)
  line L41 (3.3789, 10.45) -> (-3.3789, 10.45)
  constraint coincident L15 L17.start
  constraint coincident L0.end L1.start
  constraint perpendicular L1 L17
  constraint coincident L0.start L5.end
  constraint coincident L16 L19.end
  constraint perpendicular L16 L19
  constraint coincident L15.end L16.start
  constraint coincident L15 L22.start
  constraint coincident L1.end L2.start
  constraint coincident L2.end L3.start
  constraint coincident L14 L24.end
  constraint perpendicular L14 L24
  constraint coincident L14.end L15.start
  constraint vertical L22
  constraint coincident L4 L27.start
  constraint coincident L6.end L7.start
  constraint coincident L12 L28.end
  constraint perpendicular L27 L28
  constraint vertical L27
  constraint coincident L16 L30.end
  constraint coincident L12.start L16.end
  constraint horizontal L31
  constraint vertical L32
  constraint perpendicular L32 L33
  constraint perpendicular L33 L35
  constraint coincident L4 L32.start
  constraint coincident L9.end L10.start
  constraint coincident L13 L33.end
  constraint coincident L14 L35.end
  constraint coincident L13.end L14.start
  constraint horizontal L36
  constraint coincident L6.start L11.end
  constraint coincident L12 L37.end
  constraint perpendicular L12 L37
  constraint perpendicular L12 L39
  constraint coincident L10.end L11.start
  constraint coincident L13 L39.end
  constraint coincident L12.end L13.start
  constraint perpendicular L13 L40
extrude "押し出し2" add sketch "スケッチ2" along normal blind 15 contours L0 L15 L16 L17 L18 L19 L20 L21 | L4 L7 L12 L16 L27 L28 L29 L30 L31 | L2 L14 L15 L22 L23 L24 L25 L26 | L4 L9 L13 L14 L32 L33 L34 L35 L36 bodies 1
extrude "押し出し3" add sketch "スケッチ2" along normal blind 60 contours L11 L12 L13 L37 L38 L39 L40 L41 bodies 1
sketch "スケッチ3" plane through (0, 0, -2.5) normal (0, 0, -1) x (-1, 0, 0)
  line L0 (24.8198, 88.9909) -> (31.8909, 81.9198)
  line L1 (31.8909, 81.9198) -> (31.8909, 45.9909)
  line L2 (31.8909, 45.9909) -> (-31.8909, 45.9909)
  line L3 (-31.8909, 45.9909) -> (-31.8909, 81.9198)
  line L4 (-31.8909, 81.9198) -> (-24.8198, 88.9909)
  line L5 (-24.8198, 88.9909) -> (24.8198, 88.9909)
  line L6 (24.5921, 31.6632) -> (3.3789, 10.45)
  line L7 (3.3789, 10.45) -> (-3.3789, 10.45)
  line L8 (-3.3789, 10.45) -> (-24.5921, 31.6632)
  line L9 (-24.5921, 31.6632) -> (-24.5921, 38.8909)
  line L10 (-24.5921, 38.8909) -> (24.5921, 38.8909)
  line L11 (24.5921, 38.8909) -> (24.5921, 31.6632)
  line L12 (0, 0) -> (38.8909, 38.8909)
  line L13 (38.8909, 38.8909) -> (38.8909, 95.9909)
  line L14 (38.8909, 95.9909) -> (-38.8909, 95.9909)
  line L15 (-38.8909, 95.9909) -> (-38.8909, 38.8909)
  line L16 (-38.8909, 38.8909) -> (0, 0)
  line L17 (-38.8909, 95.9909) -> (-28.3553, 85.4553) construction
  line L18 (38.8909, 95.9909) -> (28.3553, 85.4553) construction
  circle A0 centre (-33.6231, 90.7231) radius 3.25
  circle A1 centre (33.6231, 90.7231) radius 3.25
  circle A2 centre (-31.8909, 38.8909) radius 3.25
  circle A3 centre (31.8909, 38.8909) radius 3.25
  line L19 (-24.5921, 38.8909) -> (-38.8909, 38.8909) construction
  line L20 (-31.8909, 45.9909) -> (-31.8909, 31.8909) construction
  line L21 (24.5921, 38.8909) -> (38.8909, 38.8909) construction
  line L22 (31.8909, 45.9909) -> (31.8909, 31.8909) construction
  circle A4 centre (-31.8909, 38.8909) radius 1.5
  circle A5 centre (31.8909, 38.8909) radius 1.5
  circle A6 centre (33.6231, 90.7231) radius 1.5
  circle A7 centre (-33.6231, 90.7231) radius 1.5
  dimension "d27" = 6.5
  dimension "d28" = 6.5
  dimension "d29" = 6.5
  dimension "d30" = 6.5
  dimension "d31" = 3
  dimension "d32" = 3
  dimension "d33" = 3
  dimension "d34" = 3
  constraint coincident L14.end L15.start
  constraint midpoint L4 L17.end
  constraint coincident L13.end L14.start
  constraint midpoint L0 L18.end
  constraint midpoint L17 A0.centre
  constraint midpoint L18 A1.centre
  constraint coincident L9.end L10.start
  constraint coincident L15.end L16.start
  constraint coincident L2.end L3.start
  constraint coincident L16 L20.end
  constraint perpendicular L19 L20
  constraint coincident A2.centre L19
  constraint coincident A2.centre L20
  constraint coincident L10.end L11.start
  constraint coincident L12.end L13.start
  constraint coincident L1.end L2.start
  constraint coincident L12 L22.end
  constraint perpendicular L21 L22
  constraint coincident A3.centre L22
  constraint coincident A3.centre L21
  constraint concentric A2 A4
  constraint concentric A3 A5
  constraint concentric A1 A6
  constraint concentric A0 A7
  measures "d27" diameter of A0
  measures "d28" diameter of A1
  measures "d29" diameter of A2
  measures "d30" diameter of A3
  measures "d31" diameter of A4
  measures "d32" diameter of A5
  measures "d33" diameter of A6
  measures "d34" diameter of A7
extrude "押し出し4" cut sketch "スケッチ3" against normal blind 25 contours A4 | A5 | A6 | A7 bodies 1
extrude "押し出し5" cut sketch "スケッチ3" against normal blind 15 contours A0 | A1 | A2 | A3 bodies 1
sketch "スケッチ4" plane through (0, 10.45, 0) normal (0, 1, 0) x (-1, 0, 0)
  line L0 (3.3789, -2.5) -> (3.3789, 2.5)
  line L1 (3.3789, 2.5) -> (3.3789, 62.5)
  line L2 (3.3789, 62.5) -> (-3.3789, 62.5)
  line L3 (-3.3789, 62.5) -> (-3.3789, 2.5)
  line L4 (-3.3789, 2.5) -> (-3.3789, -2.5)
  line L5 (-3.3789, -2.5) -> (3.3789, -2.5)
  arc A0 (1.5, 35) -> (-1.5, 35) centre (0, 35) ccw
  arc A1 (-1.5, 25) -> (1.5, 25) centre (0, 25) ccw
  line L6 (0, 35) -> (0, 25) construction
  line L7 (-1.5, 35) -> (-1.5, 25)
  line L8 (1.5, 35) -> (1.5, 25)
  line L9 (0, 25) -> (0, 0) construction
  dimension "d39" = 1.5
  dimension "d40" = 1.5
  dimension "d41" = 25
  dimension "d42" = 35
  constraint coincident A0.centre L6.start
  constraint coincident A1.centre L6.end
  constraint tangent A1 L8
  constraint tangent A1 L7
  constraint tangent A0 L7
  constraint coincident A1.start L7.end
  constraint vertical L7
  constraint coincident L9.end origin
  constraint vertical L9
  constraint tangent A0 L8
  measures "d39" radius of A0
  measures "d40" radius of A1
  measures "d41" vertical distance of L9.end A1.centre
  measures "d42" vertical distance of L9.end A0.centre
extrude "押し出し6" cut sketch "スケッチ4" against normal blind 4 contours A0 A1 L7 L8 bodies 1
sketch "スケッチ5" plane through (0, 0, -2.5) normal (0, 0, -1) x (-1, 0, 0)
  line L0 (24.8198, 88.9909) -> (31.8909, 81.9198)
  line L1 (31.8909, 81.9198) -> (31.8909, 45.9909)
  line L2 (31.8909, 45.9909) -> (-31.8909, 45.9909)
  line L3 (-31.8909, 45.9909) -> (-31.8909, 81.9198)
  line L4 (-31.8909, 81.9198) -> (-24.8198, 88.9909)
  line L5 (-24.8198, 88.9909) -> (24.8198, 88.9909)
  line L6 (24.5921, 31.6632) -> (3.3789, 10.45)
  line L7 (3.3789, 10.45) -> (-3.3789, 10.45)
  line L8 (-3.3789, 10.45) -> (-24.5921, 31.6632)
  line L9 (-24.5921, 31.6632) -> (-24.5921, 38.8909)
  line L10 (-24.5921, 38.8909) -> (24.5921, 38.8909)
  line L11 (24.5921, 38.8909) -> (24.5921, 31.6632)
  line L12 (0, 0) -> (38.8909, 38.8909)
  line L13 (38.8909, 38.8909) -> (38.8909, 95.9909)
  line L14 (38.8909, 95.9909) -> (-38.8909, 95.9909)
  line L15 (-38.8909, 95.9909) -> (-38.8909, 38.8909)
  line L16 (-38.8909, 38.8909) -> (0, 0)
  circle A0 centre (31.8909, 38.8909) radius 3.25
  circle A1 centre (-33.6231, 90.7231) radius 3.25
  circle A2 centre (33.6231, 90.7231) radius 3.25
  circle A3 centre (-31.8909, 38.8909) radius 3.25
  line L17 (-11.25, 45.9909) -> (-11.25, 59.4909)
  line L18 (-11.25, 59.4909) -> (11.25, 59.4909)
  line L19 (11.25, 59.4909) -> (11.25, 45.9909)
  line L20 (-17.25, 45.9909) -> (-17.25, 65.4909)
  line L21 (-17.25, 65.4909) -> (17.25, 65.4909)
  line L22 (17.25, 65.4909) -> (17.25, 45.9909)
  line L23 (0, 0) -> (0, 59.4909) construction
  circle A4 centre (-7.9, 62.4909) radius 1.5
  circle A5 centre (7.9, 62.4909) radius 1.5
  line L24 (-7.9, 62.4909) -> (7.9, 62.4909) construction
  line L25 (0, 59.4909) -> (0, 62.4909) construction
  dimension "d45" = 6
  dimension "d46" = 6
  dimension "d47" = 6
  dimension "d48" = 22.5
  dimension "d49" = 13.5
  dimension "d50" = 15.8
  dimension "d51" = 3
  dimension "d52" = 3
  dimension "d53" = 3
  constraint coincident L2 L17.start
  constraint coincident L2 L19.end
  constraint vertical L19
  constraint horizontal L18
  constraint vertical L17
  constraint coincident L2 L20.start
  constraint perpendicular L2 L20
  constraint perpendicular L20 L21
  constraint coincident L2 L22.end
  constraint perpendicular L2 L22
  constraint coincident L12.start L16.end
  constraint coincident L18 L23.end
  constraint vertical L23
  constraint midpoint L18 L23.end
  constraint coincident A4.centre L24.start
  constraint coincident A5.centre L24.end
  constraint horizontal L24
  constraint coincident L24 L25.end
  constraint vertical L25
  constraint midpoint L24 L25.end
  measures "d45" distance of L18 L21
  measures "d46" distance of L19 L22
  measures "d47" distance of L17 L20
  measures "d48" distance of L17.end L18.end
  measures "d49" distance of L17.start L17.end
  measures "d50" distance of A4.centre A5.centre
  measures "d51" distance of L23.end L25.end
  measures "d52" diameter of A4
  measures "d53" diameter of A5
extrude "押し出し7" add sketch "スケッチ5" against normal blind 5 contours L2 L17 L18 L19 L20 L21 L22 bodies 1